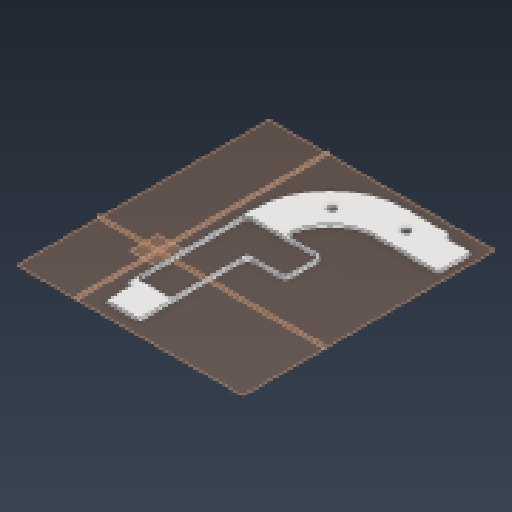
# Autodesk Inventor part: Проставка_платформы_и_столба
Saved by Autodesk Inventor 2023.2 (Build 272271030, 271C)
## iProperties
Created: 2025-10-06
Part Number: Проставка_платформы_и_столба
Material: Типовые
Document SubType Name: Modeling
Designer: Олег Коноваленко
Density: 1 g/cm^3
Appearance: По умолчанию
Author: Олег Коноваленко
Autodesk Inventor part; units mm, degrees
ref_plane "РабПлоскость1" through (0, 1.25, 0) normal (0, 1, 0) x (1, 0, 0)
sketch "Эскиз2" plane through (0, 1.25, 0) normal (0, 1, 0) x (1, 0, 0)
  arc A0 (70, 125) -> (10, 65) centre (70, 65) ccw projected
  line L0 (105, 125) -> (105, 121) projected
  line L1 (105, 121) -> (125, 121) projected
  line L2 (125, 95) -> (75, 95) projected
  line L3 (125, -125) -> (125, 125) projected
  arc A1 (75, 95) -> (40.4895, 65.8333) centre (75, 60) ccw projected
  arc A2 (40.4895, 65.8333) -> (45.4196, 60) centre (45.4196, 65) ccw projected
  line L4 (45.4196, 60) -> (65, 60) projected
  arc A3 (70, 55) -> (65, 60) centre (65, 55) ccw projected
  line L5 (70, 55) -> (70, 35) projected
  line L6 (125, 125) -> (-125, 125) projected
  line L7 (10, -35) -> (10, 65) projected
  line L8 (40, 25) -> (40, -55) projected
  arc A4 (45, 30) -> (40, 25) centre (45, 25) ccw projected
  line L9 (65, 30) -> (45, 30) projected
  arc A5 (65, 30) -> (70, 35) centre (65, 35) ccw projected
  line L10 (14, -35) -> (10, -35) projected
  line L11 (14, -55) -> (14, -35) projected
  line L12 (40, -55) -> (14, -55) projected
  circle A6 centre (25, -15) radius 3.1 projected
  circle A7 centre (25, 15) radius 3.1 projected
  circle A8 centre (25, 45) radius 3.1 projected
  circle A9 centre (55, 45) radius 3.1 projected
  circle A10 centre (40.7268, 96.1423) radius 3.05 projected
  circle A11 centre (85, 110) radius 3.1 projected
  point P0 (0, 0)
extrude "Выдавливание2" add sketch "Эскиз2" along normal mid plane 2.5 contours L6 L0 L1 L3 L2 A1 A2 L4 A3 L5 A5 L9 A4 L8 L12 L11 L10 L7 A0
sketch "Эскиз3" plane through (0, 2.5, 0) normal (0, 1, 0) x (1, 0, 0)
  line L0 (65.5, 58) -> (14.5, 58) projected
  arc A0 (14.5, 58) -> (12, 55.5) centre (14.5, 55.5) ccw projected
  line L1 (12, 55.5) -> (12, -25.5) projected
  arc A1 (68, 55.5) -> (65.5, 58) centre (65.5, 55.5) ccw projected
  line L2 (68, 34.5) -> (68, 55.5) projected
  arc A2 (65.5, 32) -> (68, 34.5) centre (65.5, 34.5) ccw projected
  line L3 (40.5, 32) -> (65.5, 32) projected
  arc A3 (40.5, 32) -> (38, 29.5) centre (40.5, 29.5) ccw projected
  line L4 (38, -25.5) -> (38, 29.5) projected
  arc A4 (35.5, -28) -> (38, -25.5) centre (35.5, -25.5) ccw projected
  line L5 (14.5, -28) -> (35.5, -28) projected
  arc A5 (12, -25.5) -> (14.5, -28) centre (14.5, -25.5) ccw projected
  point P0 (0, 0)
extrude "Выдавливание3" cut sketch "Эскиз3" against normal up to next
